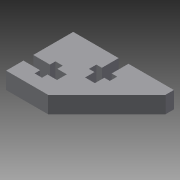
# Autodesk Inventor part: cornerBrace
Saved by Autodesk Inventor 2013 (Build 170138000, 138)
## iProperties
Created: 2014-06-23
Part Number: cornerBrace
Material: Generic
Document SubType Name: Modeling
Designer: Nano
Density: 1 g/cm^3
d0: 1.500 in
d1: 0.250 in
d2: 0.500 in
d3: 1.000 in
d4: 0.00 deg
d5: 0.875 in
Author: Nano
Autodesk Inventor part; units mm, degrees
ref_plane "YZ Plane" through (0, 0, 0) normal (1, 0, 0) x (0, 1, 0)
ref_plane "XZ Plane" through (0, 0, 0) normal (0, 1, 0) x (-1, 0, 0)
ref_plane "Work Plane1" through (0, 0, 0) normal (0, 0, 1) x (1, 0, 0)
sketch "Sketch1" plane through (0, 0, 0) normal (0, 0, 1) x (1, 0, 0)
  line L0 (41.9864, 2.5) -> (43.4368, -2.0363) construction
  arc A0 (41.9864, 2.5) -> (43.4368, -2.0363) centre (41.9864, 0) ccw construction
  line L1 (112.0586, -28.575) -> (85.0037, -28.575) construction
  line L2 (112.0586, 28.1043) -> (112.0586, -28.575) construction
  line L3 (83.2959, 28.1043) -> (112.0586, 28.1043) construction
  arc A1 (83.2959, 28.1043) -> (1.0011, 28.575) centre (41.9864, 0) ccw construction
  line L4 (-116.5414, 28.575) -> (1.0011, 28.575) construction
  line L5 (-116.5414, -29.0493) -> (-116.5414, 28.575) construction
  line L6 (-0.7121, -29.0493) -> (-116.5414, -29.0493) construction
  arc A2 (-0.7121, -29.0493) -> (85.0037, -28.575) centre (41.9864, 0) ccw construction
  line L7 (-110.1914, 28.575) -> (-110.1914, 24.0792) construction
  line L8 (-111.9045, -9.9993) -> (-73.8045, -9.9993)
  line L9 (-73.8045, -9.9993) -> (-73.8045, -16.3493)
  line L10 (-73.8045, -16.3493) -> (-111.9045, -16.3493)
  line L11 (-111.9045, -16.3493) -> (-111.9045, -9.9993)
  circle A3 centre (88.3718, 12.2257) radius 1.8542 projected
  circle A4 centre (108.8836, -22.6993) radius 1.8542 projected
  circle A5 centre (-92.8545, -12.7) radius 1.8542 projected
  circle A6 centre (-113.3664, 22.225) radius 1.8542 projected
  circle A7 centre (-92.8545, 12.2257) radius 1.8542 projected
  circle A8 centre (-113.3664, -22.6993) radius 1.8542 projected
  circle A9 centre (88.3718, -12.7) radius 1.8542 projected
  circle A10 centre (108.8836, 22.225) radius 1.8542 projected
  point P0 (0, 0)
  dimension "d0" = 38.1
  dimension "d1" = 6.35
  dimension "d2" = 12.7
  constraints: 8 end point, 2 parallel, 1 horizontal, 1 perpendicular, 1 other
  measures "d0" distance of L9.end L10.end
  measures "d1" distance of L8.end L9.end
extrude "Extrusion1" add sketch "Sketch1" along normal blind 25.4 contours L8 L9 L10 L11 | A5
chamfer "Chamfer1" distance 22.225 angle 45 1 edges at (-73.8045, -13.1743, 25.4)
sketch "Sketch2" plane through (-111.9045, -16.3493, 0) normal (0, -1, 0) x (1, 0, 0)
  line L0 (38.1, 0) -> (0, 0) projected
  line L1 (17.1958, 0) -> (20.9042, 0) projected
  line L2 (19.05, 12.7239) -> (19.05, -0.6753) construction
  line L3 (17.1958, 12.7) -> (20.9042, 12.7)
  line L4 (20.9042, 12.7) -> (20.9042, 0)
  line L5 (20.9042, 0) -> (17.1958, 0)
  line L6 (17.1958, 0) -> (17.1958, 12.7)
  line L7 (15.113, 9.144) -> (22.987, 9.144)
  line L8 (22.987, 9.144) -> (22.987, 6.35)
  line L9 (22.987, 6.35) -> (15.113, 6.35)
  line L10 (15.113, 6.35) -> (15.113, 9.144)
  line L11 (0, 0) -> (0, 25.4) projected
  line L12 (12.7, 18.8338) -> (12.7, 15.1254)
  line L13 (12.7, 15.1254) -> (0, 15.1254)
  line L14 (0, 18.8338) -> (12.7, 18.8338)
  line L15 (9.0991, 20.9166) -> (9.0991, 13.0426)
  line L16 (9.0991, 13.0426) -> (6.3051, 13.0426)
  line L17 (6.3051, 13.0426) -> (6.3051, 20.9166)
  line L18 (6.3051, 20.9166) -> (9.0991, 20.9166)
  point P0 (111.9045, 0)
  dimension "d8" = 7.874
  dimension "d9" = 2.794
  dimension "d10" = 3.937
  dimension "d11" = 3.937
  dimension "d12" = 1.9733
  dimension "d13" = 1.9733
  dimension "d14" = 6.35
  dimension "d15" = 12.7
  constraints: 32 end point, 4 parallel, 2 horizontal, 2 perpendicular, 2 point on line
  measures "d8" distance of L8.end L9.end
  measures "d9" distance of L7.end L8.end
  measures "d10" distance between parallel lines of L2 L10
  measures "d11" distance between parallel lines of L8 L2
  measures "d12" distance of L1.end L2.end
  measures "d13" distance of L1.start L2.end
  measures "d14" distance between parallel lines of L0 L9
  measures "d15" distance between parallel lines of L0 L3
extrude "Extrusion2" cut sketch "Sketch2" against normal through all
equation "\"d10\" = d11"
equation "\"d13\" = d12"
body "Solid1"
